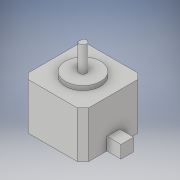
# Autodesk Inventor part: stepper motor
Saved by Autodesk Inventor 2019.3 (Build 233278000, 278)
## iProperties
Created: 2019-05-21
Part Number: stepper motor
Material: Generic
Document SubType Name: Modeling
Designer: Frienddo
Density: 1 g/cm^3
Appearance: Default
Author: Frienddo
Autodesk Inventor part; units mm, degrees
ref_plane "YZ Plane" through (0, 0, 0) normal (1, 0, 0) x (0, 1, 0)
ref_plane "XZ Plane" through (0, 0, 0) normal (0, 1, 0) x (-1, 0, 0)
ref_plane "XY Plane" through (0, 0, 0) normal (0, 0, 1) x (1, 0, 0)
sketch "Sketch1" plane through (0, 0, 0) normal (0, 1, 0) x (-1, 0, 0)
  line L0 (-21.5, -21.5) -> (21.5, -21.5)
  line L1 (21.5, -21.5) -> (21.5, 21.5)
  line L2 (21.5, 21.5) -> (-21.5, 21.5)
  line L3 (-21.5, 21.5) -> (-21.5, -21.5)
  line L4 (-21.5, -21.5) -> (21.5, 21.5) construction
  line L5 (21.5, -21.5) -> (-21.5, 21.5) construction
  point P0 (0, 0)
  dimension "d0" = 43
  dimension "d1" = 43
  constraints: 12 end point, 2 midpoint, 2 parallel, 1 horizontal, 1 perpendicular
  measures "d0" distance of L0.end L1.end
  measures "d1" distance of L1.end L2.end
extrude "Extrusion1" add sketch "Sketch1" along normal blind 33
sketch "Sketch2" plane through (21.5, 0, 21.5) normal (1, 0, 0) x (0, 0, -1)
  line L0 (43, 0) -> (0, 0) projected
  line L1 (26, 9) -> (17, 9)
  line L2 (17, 9) -> (17, 0)
  line L3 (17, 0) -> (26, 0)
  line L4 (26, 0) -> (26, 9)
  line L5 (26, 9) -> (17, 0) construction
  line L6 (17, 9) -> (26, 0) construction
  point P0 (21.5, 0)
  point P1 (21.5, 4.5)
  point P2 (21.5, 4.5)
  point P3 (21.5, 0)
  dimension "d4" = 9
  dimension "d5" = 9
  constraints: 12 end point, 4 midpoint, 2 parallel, 1 horizontal, 1 perpendicular, 1 point on line, 1 vertical alignment
  measures "d4" distance of L1.end L2.end
  measures "d5" distance of L1.start L1.end
extrude "Extrusion2" add sketch "Sketch2" along normal blind 10
chamfer "Chamfer1" distance 4 angle 45 4 edges at (21.5, 16.5, 21.5) (21.5, 16.5, -21.5) (-21.5, 16.5, 21.5) (-21.5, 16.5, -21.5)
sketch "Sketch3" plane through (0, 33, 0) normal (0, 1, 0) x (1, 0, 0)
  circle A0 centre (0, 0) radius 12.5
  line L0 (17.5, 21.5) -> (-17.5, 21.5) projected
  point P0 (0, 12.5)
  point P1 (0, -12.5)
  point P2 (0, 21.5)
  dimension "d11" = 9
  constraints: 2 point on circle, 1 centre point, 1 coincident, 1 midpoint, 1 vertical alignment
  measures "d11" distance from line of L0 A0.start
extrude "Extrusion3" add sketch "Sketch3" along normal blind 3
sketch "Sketch4" plane through (0, 36, 0) normal (0, 1, 0) x (1, 0, 0)
  arc A0 (-2, 1.5819) -> (-2, -1.5819) centre (0, 0) ccw
  line L0 (-2, -1.5819) -> (-2, 1.5819)
  arc A1 (-2, -1.5819) -> (-2, 1.5819) centre (0, 0) ccw
  point P0 (2.55, 0)
  dimension "d14" = 5.1
  dimension "d15" = 4.55
  constraints: 5 point on circle, 2 centre point, 2 end point, 1 coincident, 1 vertical
  measures "d14" diameter of A0
  measures "d15" distance from line of point (2.55, 0) L0
extrude "Extrusion4" add sketch "Sketch4" along normal blind 18 contours A1 L0
body "Solid1"
